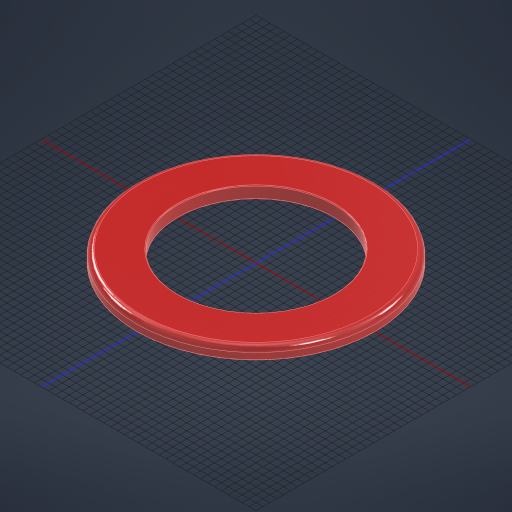
# Autodesk Inventor part: Surround
Saved by Autodesk Inventor 2023.2 (Build 272271030, 271C)
## iProperties
Created: 2023-02-22
Part Number: Surround
Material: Generisch
Document SubType Name: Modeling
Designer: Stefan
Mass: 7426.07 g
Surface Area: 5377.23 cm^2
Volume: 7426.07 cm^3
Density: 1 g/cm^3
Appearance: Rot
Author: Stefan
Autodesk Inventor part; units mm, degrees
ref_plane "YZ Plane" through (0, 0, 0) normal (1, 0, 0) x (0, 1, 0)
ref_plane "XZ Plane" through (0, 0, 0) normal (0, 1, 0) x (-1, 0, 0)
ref_plane "XY Plane" through (0, 0, 0) normal (0, 0, 1) x (1, 0, 0)
sketch "Skizze1" plane through (0, 0, 0) normal (0, 1, 0) x (-1, 0, 0)
  circle A0 centre (0, 0) radius 225.5
  circle A1 centre (0, 0) radius 345.5
  dimension "d0" = 120
  dimension "d1" = 451
  constraints: 2 centre point, 2 coincident
  measures "d0" radial gap between concentric circles of A0 A1
  measures "d1" diameter of A0
extrude "Extrusion1" add sketch "Skizze1" along normal blind 35
fillet "Rundung1" radius 15 1 edges at (345.5, 35, 0)
fillet "Rundung2" radius 2 1 edges at (225.5, 35, 0)
fillet "Rundung3" radius 2 2 edges at (345.5, 0, 0) (225.5, 0, 0)
